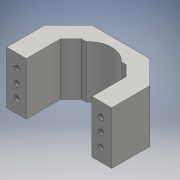
# Autodesk Inventor part: Soutient_Mot
Saved by Autodesk Inventor 2016 (Build 200138000, 138)
## iProperties
Created: 2016-05-25
Part Number: Soutient_Mot
Material: Générique
Document SubType Name: Modeling
Designer: LogOut
Density: 1 g/cm^3
Appearance: Par défaut
Author: LogOut
Autodesk Inventor part; units mm, degrees
ref_plane "YZ Plane" through (0, 0, 0) normal (1, 0, 0) x (0, 1, 0)
ref_plane "XZ Plane" through (0, 0, 0) normal (0, 1, 0) x (-1, 0, 0)
ref_plane "XY Plane" through (0, 0, 0) normal (0, 0, 1) x (1, 0, 0)
sketch "Esquisse1" plane through (0, 0, 0) normal (0, 0, 1) x (1, 0, 0)
  line L0 (-40, 30) -> (40, 30)
  line L1 (40, 30) -> (40, -17)
  line L2 (40, -17) -> (-40, -17)
  line L3 (-40, -17) -> (-40, 30)
  point P0 (0, 0)
  dimension "d0" = 47
  dimension "d1" = 80
  dimension "d2" = 40
  dimension "d3" = 30
  constraints: 8 end point, 2 parallel, 1 horizontal, 1 perpendicular
  measures "d0" distance between parallel lines of L2 L0
  measures "d1" distance of L0.start L0.end
  measures "d2" distance from line of point (0, 0) L3
  measures "d3" distance from line of point (0, 0) L0
extrude "Extrusion1" add sketch "Esquisse1" along normal blind 40
sketch "Esquisse2" plane through (0, 0, 40) normal (0, 0, 1) x (1, 0, 0)
  circle A0 centre (0, 5) radius 18
  line L0 (40, -17) -> (40, 30) projected
  line L1 (-40, 30) -> (40, 30) projected
  point P0 (0, 0)
  dimension "d6" = 36
  dimension "d7" = 40
  dimension "d8" = 25
  constraints: 1 centre point
  measures "d6" diameter of A0
  measures "d7" distance from line of L0 A0.centre
  measures "d8" distance from line of L1 A0.centre
extrude "Extrusion2" cut sketch "Esquisse2" against normal blind 40
sketch "Esquisse3" plane through (0, 0, 40) normal (0, 0, 1) x (1, 0, 0)
  circle A0 centre (0, 5) radius 18 projected
  line L0 (40, -17) -> (-40, -17) projected
  line L1 (-25, -17) -> (25, -17)
  line L2 (25, -17) -> (25, 9)
  line L3 (-25, 9) -> (-25, -17)
  line L4 (-25, 9) -> (-17, 17)
  line L5 (17, 17) -> (25, 9)
  line L6 (17, 17) -> (13.4164, 17)
  line L7 (-13.4164, 17) -> (-17, 17)
  point P0 (0, 0)
  point P1 (25, 17)
  point P2 (-25, 17)
  constraints: 14 end point, 3 parallel, 3 point on line, 2 point on circle, 1 horizontal, 1 perpendicular
extrude "Extrusion3" cut sketch "Esquisse3" against normal blind 40
sketch "Esquisse4" plane through (-40, -17, 0) normal (0, -1, 0) x (1, 0, 0)
  line L0 (8, 10) -> (72, 10)
  line L1 (72, 10) -> (72, 30)
  line L2 (72, 30) -> (8, 30)
  line L3 (8, 30) -> (8, 10)
  line L4 (0, 40) -> (80, 40) projected
  line L5 (80, 0) -> (0, 0) projected
  point P0 (40, 0)
  point P1 (15, 40)
  point P2 (65, 0)
  dimension "d23" = 64
  dimension "d24" = 32
  dimension "d25" = 10
  dimension "d26" = 10
  constraints: 8 end point, 2 parallel, 1 horizontal, 1 perpendicular
  measures "d23" distance of L0.start L0.end
  measures "d24" distance from line of point (40, 0) L3
  measures "d25" distance between parallel lines of L4 L2
  measures "d26" distance between parallel lines of L5 L0
hole "Perçage1" at (-32, -17, 30) at (32, -17, 30) at (32, -17, 10) at (-32, -17, 10) direction (0, 1, 0) diameter 4 depth 100 tip angle 118
sketch "Esquisse5" plane through (-40, 30, 0) normal (0, 1, 0) x (1, 0, 0)
  circle A0 centre (72, -30) radius 2 projected
  line L0 (8, -10) -> (72, -10)
  line L1 (72, -10) -> (72, -30)
  line L2 (72, -30) -> (8, -30)
  line L3 (8, -30) -> (8, -10)
  circle A1 centre (8, -10) radius 2 projected
  line L4 (8, -20) -> (72, -20)
  point P0 (40, 0)
  constraints: 10 end point, 2 midpoint, 2 parallel, 1 coincident, 1 horizontal, 1 perpendicular
hole "Perçage2" at (-32, 30, 10) at (-32, 30, 20) at (-32, 30, 30) at (32, 30, 30) at (32, 30, 20) at (32, 30, 10) direction (0, -1, 0) diameter 4 depth 100 tip angle 118 counterbore diameter 6 counterbore depth 43
chamfer "Chanfrein2" distance 18 distance2 18 1 edges at (40, 30, 20)
chamfer "Chanfrein3" distance 18 distance2 18 1 edges at (-40, 30, 20)
